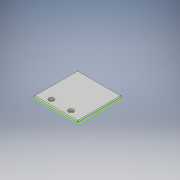
# Autodesk Inventor part: ohisje_pokrov
Saved by Autodesk Inventor 2019 (Build 230136000, 136)
## iProperties
Created: 2020-07-23
Part Number: ohisje_pokrov
Material: Generic
Document SubType Name: Modeling
Designer: lukad
Density: 1 g/cm^3
Appearance: Default
Author: lukad
Autodesk Inventor part; units mm, degrees
ref_plane "YZ Plane" through (0, 0, 0) normal (1, 0, 0) x (0, 1, 0)
ref_plane "XZ Plane" through (0, 0, 0) normal (0, 1, 0) x (-1, 0, 0)
ref_plane "XY Plane" through (0, 0, 0) normal (0, 0, 1) x (1, 0, 0)
sketch "Sketch2" plane through (0, 0, 0) normal (0, 1, 0) x (-1, 0, 0)
  line L0 (9.0054, 31.9458) -> (-44.9946, 31.9458)
  line L1 (-44.9946, 31.9458) -> (-44.9946, -22.0542)
  line L2 (-44.9946, -22.0542) -> (9.0054, -22.0542)
  line L3 (9.0054, -22.0542) -> (9.0054, 31.9458)
  line L4 (7.0054, 29.9458) -> (-42.9946, 29.9458)
  line L5 (-42.9946, 29.9458) -> (-42.9946, -20.0542)
  line L6 (-42.9946, -20.0542) -> (7.0054, -20.0542)
  line L7 (7.0054, -20.0542) -> (7.0054, 29.9458)
  line L8 (6.0054, 28.9458) -> (-41.9946, 28.9458)
  line L9 (-41.9946, 28.9458) -> (-41.9946, -19.0542)
  line L10 (-41.9946, -19.0542) -> (6.0054, -19.0542)
  line L11 (6.0054, -19.0542) -> (6.0054, 28.9458)
  circle A0 centre (-5.9946, 24.9458) radius 3.05
  circle A1 centre (-5.9946, 24.9458) radius 4
  line L12 (-17.9946, 28.9458) -> (-17.9946, -19.0542)
  circle A2 centre (-29.9946, 24.9458) radius 3.05
  circle A3 centre (-29.9946, 24.9458) radius 4
  point P0 (0, 0)
  dimension "d8" = 54
  dimension "d9" = 2
  dimension "d10" = 2
  dimension "d11" = 2
  dimension "d12" = 2
  dimension "d13" = 48
  dimension "d14" = 1
  dimension "d15" = 1
  dimension "d16" = 1
  dimension "d17" = 1
  dimension "d24" = 50
  dimension "d25" = 6.1
  dimension "d26" = 12
  dimension "d28" = 8
  dimension "d29" = 25
  dimension "d30" = 25
  dimension "d39" = 5
  constraints: 26 end point, 7 perpendicular, 6 parallel, 4 centre point, 3 horizontal, 2 coincident, 2 midpoint, 2 symmetric about line, 2 other
  measures "d8" distance of L2.end L1.end
  measures "d9" distance between parallel lines of L3 L7
  measures "d10" distance between parallel lines of L1 L5
  measures "d11" distance between parallel lines of L2 L6
  measures "d12" distance between parallel lines of L0 L4
  measures "d13" distance between parallel lines of L10 L8
  measures "d14" distance between parallel lines of L7 L11
  measures "d15" distance between parallel lines of L9 L5
  measures "d16" distance between parallel lines of L4 L8
  measures "d17" distance between parallel lines of L6 L10
  measures "d24" distance between parallel lines of L6 L4
  measures "d25" diameter of A0
  measures "d26" distance from line of A0.centre L11
  measures "d28" diameter of A1
  measures "d29" distance between parallel lines of L5 L12
  measures "d30" distance between parallel lines of L7 L12
  measures "d39" distance from line of A0.centre L4
extrude "Extrusion1" add sketch "Sketch2" along normal blind 2 contours L3 L2 L1 L0 | L7 L6 L5 L4 | A1 | L11 L10 L12 L8 | A3 | L12 L10 L9 L8 | A0 | A2
extrude "Extrusion2" add sketch "Sketch2" against normal blind 2 contours L7 L6 L5 L4
fillet "Fillet1" radius 1 4 edges at (17.9946, 2, -22.0542) (44.9946, 2, 4.9458) (17.9946, 2, 31.9458) (-9.0054, 2, 4.9458)
fillet "Fillet2" radius 1 8 edges at (-9.0054, 0.5, 31.9458) (-8.7125, 1.7071, 31.6529) (-9.0054, 0.5, -22.0542) (-8.7125, 1.7071, -21.7613) (44.9946, 0.5, -22.0542) (44.7017, 1.7071, -21.7613) (44.9946, 0.5, 31.9458) (44.7017, 1.7071, 31.6529)
extrude "Extrusion3" cut sketch "Sketch2" along normal blind 2 contours A0
extrude "Extrusion4" cut sketch "Sketch2" along normal blind 2 contours A2
extrude "Extrusion5" add sketch "Sketch2" against normal blind 1 contours A3
extrude "Extrusion6" add sketch "Sketch2" against normal blind 1 contours A1
body "Solid1"
